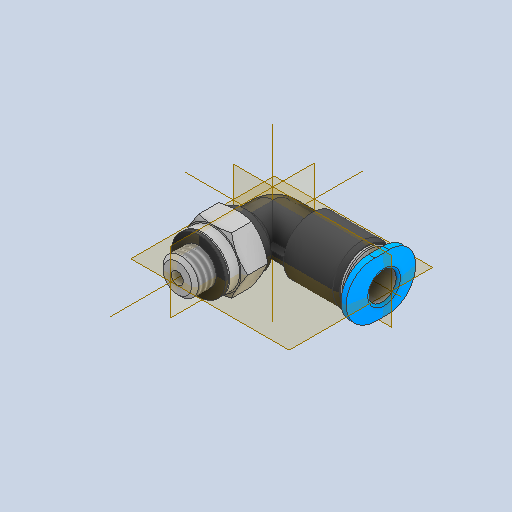
# Autodesk Inventor part: 153333 QSML-M5-4
Saved by Autodesk Inventor 2025.2 (Build 292293000, 293)
## iProperties
Category: PARTsolutions
Company: FESTO
Created: 2025-06-05
Part Number: 153333 QSML-M5-4
Material: Generic
Catalog Web Link: www.cadenas.de
Description: QSML-push-in L-fitting
Vendor: FESTO
Document SubType Name: Modeling
Designer: psAdmin
Manufacturer: FESTO
Mass: 3.4 g
Surface Area: 11.0208 cm^2
Volume: 0.948954 cm^3
Density: 1 g/cm^3
Appearance: PSOLRGB-175-175-175
PSOL_IDENT_0: {$CADENAS_DATA/23d-libs/festo/parts/q/qsml/qsml.prj},170 {VTYP=3D},{NB=153333 QSML-M5-4},{LINA=15333
PSOL_IDENT_1: 3 QSML-M5-4},{NN=QSML},{DATE=02.05.2025 12:43:59},{GEOMDATE=01.04.2025 10:00:42},{VERSION=},{LINEID=
PSOL_IDENT_2: 40},{WBVAR=},{WBNUMERIC=}  {NB=153333 QSML-M5-4},{LINA=153333 QSML-M5-4},{KT=1},{TNR=153333},{TYP=QS
PSOL_IDENT_3: ML-M5-4},{FDT=1},{FDTQS=46},{FDTQS1=34},{FDTQS2=46},{FDTQSDZX=46},{ZOLL=5},{ZOLLDRVS=5},{ZOLLDFM=5},
PSOL_IDENT_4: {ZOLLDFMCN=5},{ZOLLAXNS=5},{ZOLLDZX=5},{D=M5},{D1=4},{D2=8.000},{H=13.500},{H1=3.000},{H2=0.000},{L=
PSOL_IDENT_5: 15.700},{SW=8.000},{DN=5.000},{TYPE=1.000},{Z=0},{PSTOL=0.1},{C=11.600},{X=7.800},{Y=9.800},{NENN=1.
PSOL_IDENT_6: 700},{CNSMASSEXACT=0.0034},{MOM=1.33 ±0.27},{GTIN=4052568011314},{REACH=Ja},{REACHSVHC=Ja},{REACHHAZ
PSOL_IDENT_7: SUBS=7439-92-1},{REACHSCIP=4683995a-6d2d-4183-809b-b444404038eb},{REACHVALDATE=05.03.2025}
NB: 153333 QSML-M5-4
NN: QSML
NT: push-in L-fitting
NBSYN: $TNR. $TYP.
LINA: 153333 QSML-M5-4
CATALOG: Festo
TNR: 153333
TYP: QSML-M5-4
D: M5
D1: 4
D2: 8
H: 13.5
H1: 3
H2: 0
L: 15.7
SW: 8
NENN: 1.7
CNSMASSEXACT: 0.0034
MOM: 1.33 ±0.27
GTIN: 4052568011314
REACH: Yes
REACHSVHC: Yes
REACHHAZSUBS: 7439-92-1
REACHVALDATE: 05.03.2025
SUPPLIER: FESTO
ARTICLENO: 153333 QSML-M5-4
BOMINFO: 153333 QSML-M5-4
CREATOR: CADENAS GmbH
Title: 153333 QSML-M5-4
Author: Cadenas PARTsolutions
Comments: push-in L-fitting
Autodesk Inventor part; units mm, degrees
sketch "Sketch_1" plane through (0, 0, 0) normal (0, 0, 1) x (1, 0, 0)
  line L0 (15.7, 0) -> (-2.8, 0)
  arc A0 (0, 2.8) -> (-2.8, 0) centre (0, 0) ccw
  line L1 (0, 2.8) -> (4.8072, 2.8)
  line L2 (4.8072, 2.8) -> (5.5, 4)
  line L3 (5.5, 4) -> (12.4571, 4)
  line L4 (12.4571, 4) -> (13.2, 3.801)
  line L5 (13.2, 3.801) -> (13.2, 3.6938)
  line L6 (13.2, 3.6938) -> (13.4586, 3.6938)
  line L7 (13.4586, 3.6938) -> (13.6, 3.5524)
  line L8 (13.6, 3.5524) -> (13.6, 2.5)
  line L9 (13.6, 2.5) -> (14.13, 2.5)
  arc A1 (14.13, 2.5) -> (14.5, 2.87) centre (14.13, 2.87) ccw
  line L10 (14.5, 2.87) -> (14.5, 5.9)
  line L11 (14.5, 5.9) -> (14.8974, 5.9)
  arc A2 (15.0944, 5.7347) -> (14.8974, 5.9) centre (14.8974, 5.7) ccw
  line L12 (15.0944, 5.7347) -> (15.7, 2.3)
  line L13 (15.7, 2.3) -> (15.7, 0)
  line L14 (15.7, 0) -> (-2.8, 0)
  constraints: 30 end point, 6 point on circle, 3 centre point
revolve "Revolution1" add sketch "Sketch_1" angle 360 about axis through (15.7, 0, 0) along (-1, 0, 0)
sketch "Sketch_2" plane through (0, 0, 0) normal (1, 0, 0) x (0, 1, 0)
  line L0 (0, 0) -> (0, 10.5)
  line L1 (0, 10.5) -> (3.8, 10.5)
  line L2 (3.8, 10.5) -> (3.8, 10.1)
  line L3 (3.8, 10.1) -> (3.7, 10)
  line L4 (3.7, 10) -> (3.8, 9.9)
  line L5 (3.8, 9.9) -> (3.8, 8.5)
  line L6 (3.8, 8.5) -> (4, 8.5)
  line L7 (4, 8.5) -> (4.64, 8.1305)
  line L8 (4.64, 8.1305) -> (4.64, 5.3695)
  line L9 (4.64, 5.3695) -> (4, 5)
  line L10 (4, 5) -> (3.75, 5)
  line L11 (3.75, 5) -> (3.75, 4)
  line L12 (3.75, 4) -> (2.8, 3.05)
  line L13 (2.8, 3.05) -> (2.8, 0)
  line L14 (2.8, 0) -> (0, 0)
  line L15 (0, 0) -> (0, 10.5)
  constraints: 32 end point
revolve "Revolution2" add sketch "Sketch_2" angle 360 about axis through (0, 0, 0) along (0, 0, 1)
sketch "Sketch_3" plane through (0, 0, 0) normal (1, 0, 0) x (0, 1, 0)
  line L0 (0, 10.5) -> (0, 13.5)
  line L1 (0, 13.5) -> (2.0095, 13.5)
  line L2 (2.0095, 13.5) -> (2.5, 13.0095)
  line L3 (2.5, 13.0095) -> (2.5, 10.5)
  line L4 (2.5, 10.5) -> (0, 10.5)
  line L5 (0, 10.5) -> (0, 13.5)
  constraints: 12 end point
revolve "Revolution3" add sketch "Sketch_3" angle 360 about axis through (0, 0, 10.5) along (0, 0, 1)
thread "Thread1" size "M5x0.8" class "6g" standard "ISO Metric profile" full length
sketch "Sketch_11" plane through (15.7, 0, 0) normal (1, 0, 0) x (0, 0, -1)
  line L0 (-9.8, -5.658) -> (0, -11.3161)
  line L1 (0, -11.3161) -> (9.8, -5.658)
  line L2 (9.8, -5.658) -> (9.8, 5.658)
  line L3 (9.8, 5.658) -> (0, 11.3161)
  line L4 (0, 11.3161) -> (-9.8, 5.658)
  line L5 (-9.8, 5.658) -> (-9.8, -5.658)
  arc A0 (-1, 3.9) -> (-1, -3.9) centre (-1, 0) ccw
  line L6 (-1, -3.9) -> (1, -3.9)
  arc A1 (1, -3.9) -> (1, 3.9) centre (1, 0) ccw
  line L7 (1, 3.9) -> (-1, 3.9)
  constraints: 16 end point, 4 point on circle, 2 centre point
extrude "Extrusion1" cut sketch "Sketch_11" against normal blind 1.2
sketch "Sketch_5" plane through (0, 0, 0) normal (0, 1, 0) x (-1, 0, 0)
  line L0 (-15.7, 0) -> (0.85, 0)
  arc A0 (0, -0.85) -> (0.85, 0) centre (0, 0) ccw
  line L1 (0, -0.85) -> (-4.1, -0.85)
  line L2 (-4.1, -0.85) -> (-4.1, -2)
  line L3 (-4.1, -2) -> (-15.4, -2)
  arc A1 (-15.4, -2) -> (-15.7, -2.3) centre (-15.4, -2.3) ccw
  line L4 (-15.7, -2.3) -> (-15.7, 0)
  line L5 (-15.7, 0) -> (0.85, 0)
  constraints: 12 end point, 4 point on circle, 2 centre point
sketch "Sketch_15" plane through (0, 0, 0) normal (0, 1, 0) x (-1, 0, 0)
  line L0 (3.75, -1) -> (3.75, 4)
  line L1 (3.75, 4) -> (-5.5, 4)
  line L2 (-5.5, 4) -> (-5.5, -4)
  line L3 (-5.5, -4) -> (0.75, -4)
  arc A0 (0.75, -4) -> (3.75, -1) centre (0.75, -1) ccw
  constraints: 8 end point, 2 point on circle, 1 centre point
extrude "Extrusion2" add sketch "Sketch_15" along normal mid plane 1
sketch "Sketch_6" plane through (0, 0, 0) normal (1, 0, 0) x (0, 1, 0)
  line L0 (0, 0) -> (0, 13.5)
  line L1 (0, 13.5) -> (0.85, 13.5)
  line L2 (0.85, 13.5) -> (0.85, 0)
  line L3 (0.85, 0) -> (0, 0)
  line L4 (0, 0) -> (0, 13.5)
  constraints: 10 end point
revolve "Revolution4" cut sketch "Sketch_6" angle 360 about axis through (0, 0, 0) along (0, 0, 1)
revolve "Revolution5" cut sketch "Sketch_5" angle 360 about axis through (15.7, 0, 0) along (-1, 0, 0)
sketch "Sketch_9" plane through (0, 0, 10.5) normal (0, 0, 1) x (1, 0, 0)
  line L0 (-8, -8) -> (8, -8)
  line L1 (8, -8) -> (8, 8)
  line L2 (8, 8) -> (-8, 8)
  line L3 (-8, 8) -> (-8, -8)
  line L4 (-4.6188, 0) -> (-2.3094, -4)
  line L5 (-2.3094, -4) -> (2.3094, -4)
  line L6 (2.3094, -4) -> (4.6188, 0)
  line L7 (4.6188, 0) -> (2.3094, 4)
  line L8 (2.3094, 4) -> (-2.3094, 4)
  line L9 (-2.3094, 4) -> (-4.6188, 0)
  constraints: 20 end point
extrude "Extrusion3" cut sketch "Sketch_9" against normal blind 6.0556
ref_plane "ANBAU_XY" through (0, 0, 10.5) normal (0, 0, 1) x (1, 0, 0)
ref_plane "ANBAU_YZ" through (0, 0, 10.5) normal (1, 0, 0) x (0, 1, 0)
ref_plane "ANBAU_ZX" through (0, 0, 10.5) normal (0, 1, 0) x (0, 0, 1)
ref_plane "ANBAU_STD_XY" through (0, 0, 10.5) normal (0, 0, -1) x (1, 0, 0)
ref_plane "ANBAU_STD_YZ" through (0, 0, 10.5) normal (1, 0, 0) x (0, -1, 0)
ref_plane "ANBAU_STD_ZX" through (0, 0, 10.5) normal (0, -1, 0) x (0, 0, -1)
ref_plane "CPV_XY" through (0, 0, 10.5) normal (0, 0, -1) x (1, 0, 0)
ref_plane "CPV_YZ" through (0, 0, 10.5) normal (1, 0, 0) x (0, -1, 0)
ref_plane "CPV_ZX" through (0, 0, 10.5) normal (0, -1, 0) x (0, 0, -1)
ref_plane "FDT_MOUNT_XY" through (0, 0, 10.5) normal (0, 0, 1) x (0, 1, 0)
ref_plane "FDT_MOUNT_YZ" through (0, 0, 10.5) normal (0, 1, 0) x (-1, 0, 0)
ref_plane "FDT_MOUNT_ZX" through (0, 0, 10.5) normal (-1, 0, 0) x (0, 0, 1)
ref_plane "FDT_SCHLAUCH_XY" through (4.1, 0, 0) normal (1, 0, 0) x (0, 0, -1)
ref_plane "FDT_SCHLAUCH_YZ" through (4.1, 0, 0) normal (0, 0, -1) x (0, 1, 0)
ref_plane "FDT_SCHLAUCH_ZX" through (4.1, 0, 0) normal (0, 1, 0) x (1, 0, 0)
body "Solid1"
